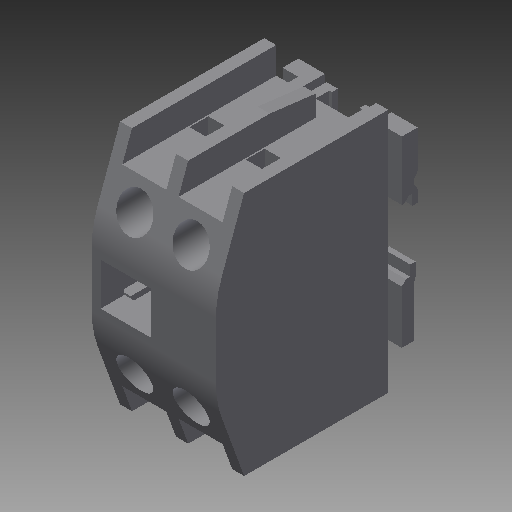
# Autodesk Inventor part: 277946
Saved by Autodesk Inventor 2019.3 (Build 233278000, 278)
## iProperties
Category: PARTsolutions
Company: MOELLER
Created: 2018-11-07
Part Number: 277946
Material: Generic
Catalog Web Link: www.cadenas.de
Description: Front mounting auxiliary contact-
Vendor: MOELLER
Document SubType Name: Modeling
Designer: psadmin
Manufacturer: MOELLER
Mass: 21.259 g
Surface Area: 127.128 cm^2
Volume: 21.259 cm^3
Density: 1 g/cm^3
Appearance: PSOLRGB-175-175-175
PSOL_IDENT_0: {$CADENAS_DATA\23d-libs\moeller\2\695\733\759\760.prj},191 {VTYP=3D},{NB=277946},{LINA=277946},{NN=F
PSOL_IDENT_1: ront mounting auxiliary contact},{DATE=04.10.2018 12:16:44},{GEOMDATE=04.10.2018 08:29:25},{VERSION=
PSOL_IDENT_2: v181004082925},{LINEID=80},{WBVAR=},{WBNUMERIC=}  {NB=277946},{LINA=277946},{KT=DUMMY},{PFOTO=2110pi
PSOL_IDENT_3: c-5.jpg},{PLID=277946},{DATA_SHEET=Data sheet},{MANUTYPEDESC=DILM150-XHI11},{DESCSHORT=Auxiliary con
PSOL_IDENT_4: tact module, 1N/O+1N/C},{DESCLONG=Top mounting auxiliary contact with interlocked opposing contacts,
PSOL_IDENT_5: tool-less mounting},{EAN=4015082779467},{ECLASS_8_1=27-37-13-02},{PACKAGED_WEIGHT=0.030},{DATA_SHEE
PSOL_IDENT_6: T_=http://datasheet.moeller.net/datasheet.php?model=277946&locale=en_GB},{DATA_SHEET_ENG=http://data
PSOL_IDENT_7: sheet.moeller.net/datasheet.php?model=277946&locale=en_GB},{DATA_SHEET_DEU=http://datasheet.moeller.
PSOL_IDENT_8: net/datasheet.php?model=277946&locale=de_DE}
NN: Front mounting auxiliary contact
NB: 277946
NBSYN: $PLID.
LINA: 277946
PFOTO: 2110pic-5.jpg
PLID: 277946
DATA_SHEET: Data sheet
MANUTYPEDESC: DILM150-XHI11
DESCSHORT: Auxiliary contact module, 1N/O+1N/C
DESCLONG: Top mounting auxiliary contact with interlocked opposing contacts, tool-less mounting
EAN: 4015082779467
ECLASS_8_1: 27-37-13-02
PACKAGED_WEIGHT: 0.03
SUPPLIER: MOELLER
ARTICLENO: 277946
BOMINFO: 277946
CREATOR: CADENAS GmbH
Title: 277946
Author: Cadenas PARTsolutions
Autodesk Inventor part; units mm, degrees
sketch "Sketch_1" plane through (0, 0, 0) normal (1, 0, 0) x (0, 1, 0)
  arc A0 (-5.3261, 32.5) -> (-11.4825, 31.4145) centre (-5.3261, 14.5) ccw
  line L0 (-11.4825, 31.4145) -> (-23.1, 27.186)
  line L1 (-23.1, 27.186) -> (-23.1, 0)
  line L2 (-23.1, 0) -> (-17.5, 0)
  line L3 (-17.5, 0) -> (-17.5, -5.35)
  line L4 (-17.5, -5.35) -> (-9.1529, -5.35)
  arc A1 (-9.1529, -5.35) -> (-8.6412, -5.26) centre (-9.1529, -3.85) ccw
  arc A2 (-7.7574, -5.36) -> (-8.6412, -5.26) centre (-8.3, -6.2) ccw
  arc A3 (-7.7574, -5.36) -> (-6.9435, -5.6) centre (-6.9435, -4.1) ccw
  line L5 (-6.9435, -5.6) -> (-4.7, -5.6)
  line L6 (-4.7, -5.6) -> (-4.7, -4.6)
  line L7 (-4.7, -4.6) -> (-6.7, -4.6)
  line L8 (-6.7, -4.6) -> (-6.7, -3.8)
  line L9 (-6.7, -3.8) -> (-7.5, -3)
  line L10 (-7.5, -3) -> (-7.7, -3)
  line L11 (-7.7, -3) -> (-7.7, 0)
  line L12 (-7.7, 0) -> (7.7, 0)
  line L13 (7.7, 0) -> (7.7, -3)
  line L14 (7.7, -3) -> (5.8314, -3)
  line L15 (5.8314, -3) -> (5.8314, -3.4243)
  line L16 (5.8314, -3.4243) -> (6.7, -4.2929)
  line L17 (6.7, -4.2929) -> (6.7, -5)
  line L18 (6.7, -5) -> (4.7, -5)
  line L19 (4.7, -5) -> (4.7, -6)
  line L20 (4.7, -6) -> (6.654, -6)
  arc A4 (6.654, -6) -> (7.7538, -5.52) centre (6.654, -4.5) ccw
  arc A5 (9.2202, -5.52) -> (7.7538, -5.52) centre (8.487, -6.2) ccw
  arc A6 (9.2202, -5.52) -> (10.32, -6) centre (10.32, -4.5) ccw
  line L21 (10.32, -6) -> (17, -6)
  line L22 (17, -6) -> (17, 0)
  line L23 (17, 0) -> (23.1, 0)
  line L24 (23.1, 0) -> (23.1, 27.186)
  line L25 (23.1, 27.186) -> (11.4825, 31.4145)
  arc A7 (11.4825, 31.4145) -> (5.3261, 32.5) centre (5.3261, 14.5) ccw
  line L26 (5.3261, 32.5) -> (-5.3261, 32.5)
  constraints: 54 end point, 16 point on circle, 8 centre point
extrude "Extrusion1" add sketch "Sketch_1" along normal blind 23.4
sketch "Sketch_2" plane through (0, 0, 0) normal (0, 1, 0) x (-1, 0, 0)
  line L0 (5, -11) -> (5, 0)
  line L1 (5, 0) -> (-3.4, 0)
  line L2 (-3.4, 0) -> (-3.4, -3)
  line L3 (-3.4, -3) -> (-0.45, -3)
  line L4 (-0.45, -3) -> (-0.45, -9)
  line L5 (-0.45, -9) -> (-6.95, -9)
  line L6 (-6.95, -9) -> (-6.95, -4.8)
  line L7 (-6.95, -4.8) -> (-16.45, -4.8)
  line L8 (-16.45, -4.8) -> (-16.45, -9)
  line L9 (-16.45, -9) -> (-22.95, -9)
  line L10 (-22.95, -9) -> (-22.95, -3)
  line L11 (-22.95, -3) -> (-20, -3)
  line L12 (-20, -3) -> (-20, 0)
  line L13 (-20, 0) -> (-28.4, 0)
  line L14 (-28.4, 0) -> (-28.4, -11)
  line L15 (-28.4, -11) -> (5, -11)
  constraints: 32 end point
extrude "Extrusion2" cut sketch "Sketch_2" along normal mid plane 46.8
sketch "Sketch_3" plane through (0, 0, 0) normal (0, 0, 1) x (1, 0, 0)
  line L0 (3.4, 7.7) -> (3.4, 0)
  line L1 (3.4, 0) -> (20, 0)
  line L2 (20, 0) -> (20, 7.7)
  line L3 (20, 7.7) -> (17.95, 7.7)
  line L4 (17.95, 7.7) -> (17.95, 23.1)
  line L5 (17.95, 23.1) -> (16.45, 23.1)
  line L6 (16.45, 23.1) -> (16.45, 7.7)
  line L7 (16.45, 7.7) -> (6.95, 7.7)
  line L8 (6.95, 7.7) -> (6.95, 23.1)
  line L9 (6.95, 23.1) -> (5.45, 23.1)
  line L10 (5.45, 23.1) -> (5.45, 7.7)
  line L11 (5.45, 7.7) -> (3.4, 7.7)
  constraints: 24 end point
extrude "Extrusion3" cut sketch "Sketch_3" against normal blind 6
sketch "Sketch_27" plane through (0, 0, -6) normal (0, 0, 1) x (1, 0, 0)
  line L0 (5.45, 0) -> (5.45, -13.9762)
  line L1 (5.45, -13.9762) -> (7.8947, -23.1)
  line L2 (7.8947, -23.1) -> (15.5053, -23.1)
  line L3 (15.5053, -23.1) -> (17.95, -13.9762)
  line L4 (17.95, -13.9762) -> (17.95, 0)
  line L5 (17.95, 0) -> (5.45, 0)
  constraints: 12 end point
extrude "Extrusion4" cut sketch "Sketch_27" along normal blind 7
sketch "Sketch_4" plane through (0, 0, 0) normal (0, 0, 1) x (1, 0, 0)
  line L0 (2.25, 28.1) -> (2.25, 18.1)
  line L1 (2.25, 18.1) -> (10.55, 18.1)
  line L2 (10.55, 18.1) -> (10.55, 25.1)
  line L3 (10.55, 25.1) -> (12.85, 25.1)
  line L4 (12.85, 25.1) -> (12.85, 18.1)
  line L5 (12.85, 18.1) -> (21.15, 18.1)
  line L6 (21.15, 18.1) -> (21.15, 28.1)
  line L7 (21.15, 28.1) -> (2.25, 28.1)
  constraints: 16 end point
extrude "Extrusion5" cut sketch "Sketch_4" along normal blind 35
sketch "Sketch_5" plane through (0, 0, 0) normal (0, 0, 1) x (1, 0, 0)
  line L0 (2.25, -28.1) -> (21.15, -28.1)
  line L1 (21.15, -28.1) -> (21.15, -18.1)
  line L2 (21.15, -18.1) -> (12.85, -18.1)
  line L3 (12.85, -18.1) -> (12.85, -25.1)
  line L4 (12.85, -25.1) -> (10.55, -25.1)
  line L5 (10.55, -25.1) -> (10.55, -18.1)
  line L6 (10.55, -18.1) -> (2.25, -18.1)
  line L7 (2.25, -18.1) -> (2.25, -28.1)
  constraints: 16 end point
extrude "Extrusion6" cut sketch "Sketch_5" along normal blind 35
sketch "Sketch_6" plane through (11.7, 0, 0) normal (1, 0, 0) x (0, 0, -1)
  line L0 (-11.8, 28.1) -> (-11.8, 23.1)
  line L1 (-11.8, 23.1) -> (-3.1, 22.0318)
  line L2 (-3.1, 22.0318) -> (-3.1, 18.1)
  line L3 (-3.1, 18.1) -> (0, 18.1)
  line L4 (0, 18.1) -> (0, 12)
  line L5 (0, 12) -> (4.8, 12)
  line L6 (4.8, 12) -> (4.8, 28.1)
  line L7 (4.8, 28.1) -> (-11.8, 28.1)
  constraints: 16 end point
extrude "Extrusion7" cut sketch "Sketch_6" along normal mid plane 5.2
sketch "Sketch_7" plane through (11.7, 0, 0) normal (1, 0, 0) x (0, 0, -1)
  line L0 (0, 9.4) -> (3.4244, 9.4)
  line L1 (3.4244, 9.4) -> (3.6898, 17)
  line L2 (3.6898, 17) -> (0, 17)
  line L3 (0, 17) -> (0, 9.4)
  constraints: 8 end point
extrude "Extrusion8" cut sketch "Sketch_7" along normal mid plane 6.2
sketch "Sketch_8" plane through (0, 0, 0) normal (0, 0, 1) x (1, 0, 0)
  line L0 (1, 3.65) -> (1, -3.65)
  line L1 (1, -3.65) -> (2.8, -3.65)
  line L2 (2.8, -3.65) -> (2.8, -4.65)
  line L3 (2.8, -4.65) -> (10.85, -4.65)
  line L4 (10.85, -4.65) -> (10.85, -1.2)
  line L5 (10.85, -1.2) -> (12.55, -1.2)
  line L6 (12.55, -1.2) -> (12.55, 1.2)
  line L7 (12.55, 1.2) -> (10.85, 1.2)
  line L8 (10.85, 1.2) -> (10.85, 4.65)
  line L9 (10.85, 4.65) -> (2.8, 4.65)
  line L10 (2.8, 4.65) -> (2.8, 3.65)
  line L11 (2.8, 3.65) -> (1, 3.65)
  constraints: 24 end point
extrude "Extrusion9" cut sketch "Sketch_8" along normal blind 28
sketch "Sketch_9" plane through (0, 0, 0) normal (0, 0, 1) x (1, 0, 0)
  line L0 (12.55, -4.65) -> (20.6, -4.65)
  line L1 (20.6, -4.65) -> (20.6, -3.15)
  line L2 (20.6, -3.15) -> (22.4, -3.15)
  line L3 (22.4, -3.15) -> (22.4, 3.15)
  line L4 (22.4, 3.15) -> (20.6, 3.15)
  line L5 (20.6, 3.15) -> (20.6, 4.65)
  line L6 (20.6, 4.65) -> (12.55, 4.65)
  line L7 (12.55, 4.65) -> (12.55, -4.65)
  constraints: 16 end point
extrude "Extrusion10" cut sketch "Sketch_9" along normal blind 31.5
sketch "Sketch_10" plane through (0, 0, 32.5) normal (0, 0, 1) x (1, 0, 0)
  line L0 (1.65, -4) -> (11.15, -4)
  line L1 (11.15, -4) -> (11.15, 4)
  line L2 (11.15, 4) -> (1.65, 4)
  line L3 (1.65, 4) -> (1.65, -4)
  constraints: 8 end point
extrude "Extrusion11" cut sketch "Sketch_10" against normal blind 4.5
sketch "Sketch_15" plane through (0, 18.1, 0) normal (0, 1, 0) x (1, 0, 0)
  line L0 (2.5, -13.031) -> (2.5, -16.5691)
  line L1 (2.5, -16.5691) -> (10.3, -16.5691)
  line L2 (10.3, -16.5691) -> (10.3, -13.031)
  line L3 (10.3, -13.031) -> (2.5, -13.031)
  constraints: 8 end point
extrude "Extrusion12" cut sketch "Sketch_15" against normal blind 9.1
sketch "Sketch_16" plane through (0, 18.1, 0) normal (0, 1, 0) x (1, 0, 0)
  line L0 (13.1, -13.031) -> (13.1, -16.5691)
  line L1 (13.1, -16.5691) -> (20.9, -16.5691)
  line L2 (20.9, -16.5691) -> (20.9, -13.031)
  line L3 (20.9, -13.031) -> (13.1, -13.031)
  constraints: 8 end point
extrude "Extrusion13" cut sketch "Sketch_16" against normal blind 9.1
sketch "Sketch_17" plane through (0, -18.1, 0) normal (0, 1, 0) x (1, 0, 0)
  line L0 (2.5, -13.031) -> (2.5, -16.5691)
  line L1 (2.5, -16.5691) -> (10.3, -16.5691)
  line L2 (10.3, -16.5691) -> (10.3, -13.031)
  line L3 (10.3, -13.031) -> (2.5, -13.031)
  constraints: 8 end point
extrude "Extrusion14" cut sketch "Sketch_17" along normal blind 9.1
sketch "Sketch_18" plane through (0, -18.1, 0) normal (0, 1, 0) x (1, 0, 0)
  line L0 (13.1, -13.031) -> (13.1, -16.5691)
  line L1 (13.1, -16.5691) -> (20.9, -16.5691)
  line L2 (20.9, -16.5691) -> (20.9, -13.031)
  line L3 (20.9, -13.031) -> (13.1, -13.031)
  constraints: 8 end point
extrude "Extrusion15" cut sketch "Sketch_18" along normal blind 9.1
sketch "Sketch_11" plane through (0, 0, 16.8716) normal (0, 0, 1) x (1, 0, 0)
  circle A0 centre (6.4, 13.2) radius 3.3
  constraints: 1 centre point
extrude "Extrusion16" cut sketch "Sketch_11" along normal blind 28
sketch "Sketch_12" plane through (0, 0, 16.8716) normal (0, 0, 1) x (1, 0, 0)
  circle A0 centre (17, 13.2) radius 3.3
  constraints: 1 centre point
extrude "Extrusion17" cut sketch "Sketch_12" along normal blind 28
sketch "Sketch_13" plane through (0, 0, 16.8716) normal (0, 0, 1) x (1, 0, 0)
  circle A0 centre (6.4, -13.2) radius 3.3
  constraints: 1 centre point
extrude "Extrusion18" cut sketch "Sketch_13" along normal blind 28
sketch "Sketch_14" plane through (0, 0, 16.8716) normal (0, 0, 1) x (1, 0, 0)
  circle A0 centre (17, -13.2) radius 3.3
  constraints: 1 centre point
extrude "Extrusion19" cut sketch "Sketch_14" along normal blind 28
sketch "Sketch_19" plane through (0, 13.2, 0) normal (0, 1, 0) x (1, 0, 0)
  line L0 (6.4, -16.5691) -> (6.4, -10.5691)
  line L1 (6.4, -10.5691) -> (8.027, -10.5691)
  line L2 (8.027, -10.5691) -> (8.027, -15.5717)
  line L3 (8.027, -15.5717) -> (9.9, -15.5717)
  line L4 (9.9, -15.5717) -> (9.8127, -16.5691)
  line L5 (9.8127, -16.5691) -> (6.4, -16.5691)
  line L6 (6.4, -16.5691) -> (6.4, -10.5691)
  constraints: 14 end point
revolve "Revolution1" add sketch "Sketch_19" angle 360 about axis through (6.4, 13.2, 16.5691) along (0, 0, 1)
sketch "Sketch_20" plane through (0, 13.2, 0) normal (0, 1, 0) x (1, 0, 0)
  line L0 (17, -16.5691) -> (17, -10.5691)
  line L1 (17, -10.5691) -> (18.627, -10.5691)
  line L2 (18.627, -10.5691) -> (18.627, -15.5717)
  line L3 (18.627, -15.5717) -> (20.5, -15.5717)
  line L4 (20.5, -15.5717) -> (20.4127, -16.5691)
  line L5 (20.4127, -16.5691) -> (17, -16.5691)
  line L6 (17, -16.5691) -> (17, -10.5691)
  constraints: 14 end point
revolve "Revolution2" add sketch "Sketch_20" angle 360 about axis through (17, 13.2, 16.5691) along (0, 0, 1)
sketch "Sketch_21" plane through (0, -13.2, 0) normal (0, 1, 0) x (1, 0, 0)
  line L0 (6.4, -16.5691) -> (6.4, -10.5691)
  line L1 (6.4, -10.5691) -> (8.027, -10.5691)
  line L2 (8.027, -10.5691) -> (8.027, -15.5717)
  line L3 (8.027, -15.5717) -> (9.9, -15.5717)
  line L4 (9.9, -15.5717) -> (9.8127, -16.5691)
  line L5 (9.8127, -16.5691) -> (6.4, -16.5691)
  line L6 (6.4, -16.5691) -> (6.4, -10.5691)
  constraints: 14 end point
revolve "Revolution3" add sketch "Sketch_21" angle 360 about axis through (6.4, -13.2, 16.5691) along (0, 0, 1)
sketch "Sketch_22" plane through (0, -13.2, 0) normal (0, 1, 0) x (1, 0, 0)
  line L0 (17, -16.5691) -> (17, -10.5691)
  line L1 (17, -10.5691) -> (18.627, -10.5691)
  line L2 (18.627, -10.5691) -> (18.627, -15.5717)
  line L3 (18.627, -15.5717) -> (20.5, -15.5717)
  line L4 (20.5, -15.5717) -> (20.4127, -16.5691)
  line L5 (20.4127, -16.5691) -> (17, -16.5691)
  line L6 (17, -16.5691) -> (17, -10.5691)
  constraints: 14 end point
revolve "Revolution4" add sketch "Sketch_22" angle 360 about axis through (17, -13.2, 16.5691) along (0, 0, 1)
sketch "Sketch_23" plane through (0, 0, 16.8716) normal (0, 0, 1) x (1, 0, 0)
  circle A0 centre (6.4, 13.2) radius 4
  line L0 (4.4, 12.7) -> (5.9, 12.7)
  line L1 (5.9, 12.7) -> (5.9, 9.6)
  line L2 (5.9, 9.6) -> (6.9, 9.6)
  line L3 (6.9, 9.6) -> (6.9, 12.7)
  line L4 (6.9, 12.7) -> (8.4, 12.7)
  line L5 (8.4, 12.7) -> (8.4, 13.7)
  line L6 (8.4, 13.7) -> (6.9, 13.7)
  line L7 (6.9, 13.7) -> (6.9, 16.8)
  line L8 (6.9, 16.8) -> (5.9, 16.8)
  line L9 (5.9, 16.8) -> (5.9, 13.7)
  line L10 (5.9, 13.7) -> (4.4, 13.7)
  line L11 (4.4, 13.7) -> (4.4, 12.7)
  constraints: 24 end point, 1 centre point
extrude "Extrusion20" add sketch "Sketch_23" along normal blind 1.2
sketch "Sketch_24" plane through (0, 0, 16.8716) normal (0, 0, 1) x (1, 0, 0)
  circle A0 centre (17, 13.2) radius 4
  line L0 (15, 12.7) -> (16.5, 12.7)
  line L1 (16.5, 12.7) -> (16.5, 9.6)
  line L2 (16.5, 9.6) -> (17.5, 9.6)
  line L3 (17.5, 9.6) -> (17.5, 12.7)
  line L4 (17.5, 12.7) -> (19, 12.7)
  line L5 (19, 12.7) -> (19, 13.7)
  line L6 (19, 13.7) -> (17.5, 13.7)
  line L7 (17.5, 13.7) -> (17.5, 16.8)
  line L8 (17.5, 16.8) -> (16.5, 16.8)
  line L9 (16.5, 16.8) -> (16.5, 13.7)
  line L10 (16.5, 13.7) -> (15, 13.7)
  line L11 (15, 13.7) -> (15, 12.7)
  constraints: 24 end point, 1 centre point
extrude "Extrusion21" add sketch "Sketch_24" along normal blind 1.2
sketch "Sketch_25" plane through (0, 0, 16.8716) normal (0, 0, 1) x (1, 0, 0)
  circle A0 centre (6.4, -13.2) radius 4
  line L0 (4.4, -13.7) -> (5.9, -13.7)
  line L1 (5.9, -13.7) -> (5.9, -16.8)
  line L2 (5.9, -16.8) -> (6.9, -16.8)
  line L3 (6.9, -16.8) -> (6.9, -13.7)
  line L4 (6.9, -13.7) -> (8.4, -13.7)
  line L5 (8.4, -13.7) -> (8.4, -12.7)
  line L6 (8.4, -12.7) -> (6.9, -12.7)
  line L7 (6.9, -12.7) -> (6.9, -9.6)
  line L8 (6.9, -9.6) -> (5.9, -9.6)
  line L9 (5.9, -9.6) -> (5.9, -12.7)
  line L10 (5.9, -12.7) -> (4.4, -12.7)
  line L11 (4.4, -12.7) -> (4.4, -13.7)
  constraints: 24 end point, 1 centre point
extrude "Extrusion22" add sketch "Sketch_25" along normal blind 1.2
sketch "Sketch_26" plane through (0, 0, 16.8716) normal (0, 0, 1) x (1, 0, 0)
  circle A0 centre (17, -13.2) radius 4
  line L0 (15, -13.7) -> (16.5, -13.7)
  line L1 (16.5, -13.7) -> (16.5, -16.8)
  line L2 (16.5, -16.8) -> (17.5, -16.8)
  line L3 (17.5, -16.8) -> (17.5, -13.7)
  line L4 (17.5, -13.7) -> (19, -13.7)
  line L5 (19, -13.7) -> (19, -12.7)
  line L6 (19, -12.7) -> (17.5, -12.7)
  line L7 (17.5, -12.7) -> (17.5, -9.6)
  line L8 (17.5, -9.6) -> (16.5, -9.6)
  line L9 (16.5, -9.6) -> (16.5, -12.7)
  line L10 (16.5, -12.7) -> (15, -12.7)
  line L11 (15, -12.7) -> (15, -13.7)
  constraints: 24 end point, 1 centre point
extrude "Extrusion23" add sketch "Sketch_26" along normal blind 1.2
ref_plane "DIL_M150_XHI_2_XY" through (0, 0, 0) normal (0, 0, 1) x (1, 0, 0)
ref_plane "DIL_M150_XHI_2_YZ" through (0, 0, 0) normal (1, 0, 0) x (0, 1, 0)
ref_plane "DIL_M150_XHI_2_ZX" through (0, 0, 0) normal (0, 1, 0) x (0, 0, 1)
ref_plane "XHI__XY" through (11.7, 0, 0) normal (0, 0, 1) x (1, 0, 0)
ref_plane "XHI__YZ" through (11.7, 0, 0) normal (1, 0, 0) x (0, 1, 0)
ref_plane "XHI__ZX" through (11.7, 0, 0) normal (0, 1, 0) x (0, 0, 1)
body "Solid1"
